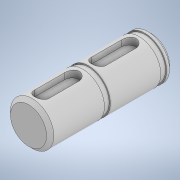
# Autodesk Inventor part: Shaft_stage_output
Saved by Autodesk Inventor 2020 (Build 240168000, 168)
## iProperties
Created: 2020-05-12
Part Number: Shaft_stage_output
Material: Generic
Document SubType Name: Sheet Metal
Designer: avi41
Density: 1 g/cm^3
Appearance: Default
Sheet Metal Rule: Default
Author: avi41
Autodesk Inventor part; units mm, degrees
ref_plane "YZ Plane" through (0, 0, 0) normal (1, 0, 0) x (0, 1, 0)
ref_plane "XY Plane" through (0, 0, 0) normal (0, 0, 1) x (1, 0, 0)
sketch "Sketch1" plane through (0, 0, 0) normal (0, 1, 0) x (-1, 0, 0)
  line L0 (0, -11.9) -> (0, 11.9) construction
  line L1 (-3.6, 0) -> (0.6, 0) construction
  line L2 (0, 8.5) -> (-3, 8.5)
  line L3 (-3, 8.5) -> (-3, -8.5)
  line L4 (-3, -8.5) -> (0, -8.5)
  line L5 (0, 8.5) -> (0, -8.5)
  point P0 (0, 0)
  dimension "d0" = 3
  dimension "d1" = 17
  constraints: 8 end point, 3 perpendicular, 2 point on line, 1 horizontal, 1 other
  measures "d0" distance of L3.end L4.end
  measures "d1" distance of L2.end L3.end
revolve "Revolution1" add sketch "Sketch1" angle 360 about axis through (0, 0, 8.5) along (0, 0, -1)
sketch "Sketch2" plane through (0, 0, 0) normal (0, 1, 0) x (-1, 0, 0)
  line L0 (0, -11.76) -> (0, 11.76) construction
  line L1 (-3, 1) -> (-2.85, 1)
  line L2 (-2.85, 1) -> (-2.85, 0.2)
  line L3 (-2.85, 0.2) -> (-3, 0.2)
  line L4 (-3, 0.2) -> (-3, 1)
  line L5 (-3, -6.8) -> (-2.85, -6.8)
  line L6 (-2.85, -6.8) -> (-2.85, -7.6)
  line L7 (-2.85, -7.6) -> (-3, -7.6)
  line L8 (-3, -7.6) -> (-3, -6.8)
  line L9 (3, -8.5) -> (-3, -8.5) projected
  line L10 (-3, -8.5) -> (-3, 8.5) projected
  dimension "d58" = 7
  dimension "d71" = 0.9
  dimension "d72" = 2.85
  dimension "d73" = 0.8
  constraints: 16 end point, 4 collinear, 4 parallel, 2 horizontal, 2 perpendicular
  measures "d58" distance from line of L5 L2.end
  measures "d71" distance between parallel lines of L9 L7
  measures "d72" distance between parallel lines of L0 L2
  measures "d73" distance of L3.end L1.start
revolve "Revolution2" cut sketch "Sketch2" angle 360 about axis through (0, 0, 0) along (0, 0, 1)
ref_plane "Work Plane2" through (0, 3, 0) normal (0, 1, 0) x (-1, 0, 0)
sketch "Sketch4" plane through (0, 3, 0) normal (0, 1, 0) x (-1, 0, 0)
  line L0 (0, -13.36) -> (0, 20.66) construction
  line L1 (1, -5.375) -> (1, -1.225)
  line L2 (-1, -1.225) -> (-1, -5.375)
  arc A0 (-1, -5.375) -> (1, -5.375) centre (0, -5.375) ccw
  arc A1 (1, -1.225) -> (-1, -1.225) centre (0, -1.225) ccw
  line L3 (3, -8.5) -> (-3, -8.5) projected
  line L4 (-1, -3.3) -> (1, -3.3) construction
  line L5 (-3, 0.2) -> (3, 0.2) construction
  line L6 (3, -6.8) -> (-3, -6.8) construction
  line L7 (3, 1) -> (-3, 1) construction
  line L8 (-3, 1) -> (-3, 8.5) projected
  line L9 (1, 6.65) -> (1, 2.5)
  line L10 (-1, 2.5) -> (-1, 6.65)
  arc A2 (1, 6.65) -> (-1, 6.65) centre (0, 6.65) ccw
  arc A3 (-1, 2.5) -> (1, 2.5) centre (0, 2.5) ccw
  line L11 (-1, 15.8) -> (1, 15.8) construction
  point P0 (0, 0)
  point P1 (-3, -1)
  point P2 (3, -1)
  dimension "d49" = 6.15
  dimension "d50" = 1
  dimension "d60" = 3.5
  dimension "d61" = 3.5
  dimension "d74" = 1
  dimension "d75" = 1
  dimension "d77" = 6.15
  dimension "d78" = 1.5
  constraints: 12 end point, 8 point on circle, 5 tangent, 4 centre point, 3 point on line, 2 midpoint, 1 parallel, 1 vertical, 2 other
  measures "d50" radius of A0
  measures "d60" distance between parallel lines of L4 L6
  measures "d61" distance between parallel lines of L5 L4
  measures "d74" radius of A3
  measures "d75" radius of A2
  measures "d78" distance from line of A3.centre L7
extrude "Extrusion2" cut sketch "Sketch4" against normal blind 1
chamfer "Chamfer3" distance 0.5 angle 45 2 edges at (-3, 0, -8.5) (-3, 0, 8.5)
equation "\"module\" = 1"
equation "\"pressure_ang\" = 30deg"
equation "\"pitch\" = 3.1416 * module"
equation "\"addendum\" = 0.45 * module"
equation "\"dedendum\" = 0.65 * module"
equation "\"tooth_depth\" = addendum + dedendum"
equation "\"addendum_mod_shaft\" = 0.45 * module"
equation "\"root_fillet_r\" = 0.16 * module"
equation "\"addendum_mod_hub\" = -addendum_mod_shaft"
equation "\"nom_space_t_hub\" = nom_tooth_t_shaft"
equation "\"nom_tooth_t_shaft\" = 2.090415"
body "Solid1"
